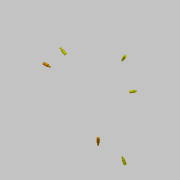
# Autodesk Inventor part: BaseAxes
Saved by Autodesk Inventor 2015 (Build 190159000, 159)
## iProperties
Created: 2016-06-12
Part Number: BaseAxes
Material: 一般
Document SubType Name: Modeling
Designer: kumagai
Density: 1 g/cm^3
Appearance: 既定
Author: kumagai
Autodesk Inventor part; units mm, degrees
ref_plane "YZ Plane" through (0, 0, 0) normal (1, 0, 0) x (0, 1, 0)
ref_plane "XZ Plane" through (0, 0, 0) normal (0, 1, 0) x (-1, 0, 0)
ref_plane "XY Plane" through (0, 0, 0) normal (0, 0, 1) x (1, 0, 0)
sketch "スケッチ1" plane through (0, 0, 0) normal (0, 1, 0) x (-1, 0, 0)
  line L0 (0, -246) -> (0, 41) projected
  line L1 (-51, 0) -> (306, 0) projected
  line L2 (255, 0) -> (255, -5)
  line L3 (255, -5) -> (235, -5)
  line L4 (235, -5) -> (235, -3)
  line L5 (235, -3) -> (225, -3)
  line L6 (225, -3) -> (225, 0)
  line L7 (255, 0) -> (225, 0)
  line L8 (0, -175) -> (0, -205)
  line L9 (3, -205) -> (0, -205)
  line L10 (3, -205) -> (3, -195)
  line L11 (3, -195) -> (5, -195)
  line L12 (5, -195) -> (5, -175)
  line L13 (5, -175) -> (0, -175)
  point P0 (0, 0)
  dimension "d0" = 30
  dimension "d1" = 30
  dimension "d2" = 10
  dimension "d3" = 10
  dimension "d4" = 5
  dimension "d5" = 5
  dimension "d6" = 3
  dimension "d7" = 3
  dimension "d8" = 195
  dimension "d9" = 235
  constraints: 24 end point, 10 perpendicular, 4 point on line, 1 vertical
  measures "d0" distance between parallel lines of L6 L2
  measures "d1" distance of L8.start L8.end
  measures "d2" distance of L4.end L5.end
  measures "d3" distance of L9.start L10.end
  measures "d4" distance of L2.start L2.end
  measures "d5" distance of L12.end L8.start
  measures "d6" distance of L5.end L6.end
  measures "d7" distance of L9.start L8.end
  measures "d8" distance from line of L1 L11.end
  measures "d9" distance from line of L0 L4.end
revolve "回転1" add sketch "スケッチ1" angle 360 about axis through (-255, 0, 0) along (1, 0, 0) contours L1 L2 L3 L4 L5 L6
revolve "回転2" add sketch "スケッチ1" angle 360 about axis through (0, 0, -175) along (0, 0, -1) contours L0 L13 L12 L11 L10 L9
pattern_circular "円形状パターン1" count 3 over 360 about axis through (0, -10, 0) along (0, 1, 0) of "回転1", "回転2"
equation "\"d0\" = ShaftLength"
equation "\"d1\" = ShaftLength"
equation "\"d2\" = ShaftInLength"
equation "\"d3\" = ShaftInLength"
equation "\"d4\" = ShaftRadius"
equation "\"d5\" = ShaftRadius"
equation "\"d6\" = ShaftInRadius"
equation "\"d7\" = ShaftInRadius"
equation "\"ShaftInRadius\" = 3"
equation "\"ShaftRadius\" = 5"
equation "\"ShaftLength\" = 30"
equation "\"ShaftInLength\" = 10"
